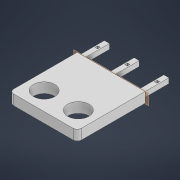
# Autodesk Inventor part: Ultrasonic Mount
Saved by Autodesk Inventor 2022 (Build 260153000, 153)
## iProperties
Created: 2021-06-09
Part Number: Ultrasonic Mount
Material: Generic
Document SubType Name: Modeling
Designer: saatvik123
Density: 1 g/cm^3
Appearance: Default
Author: saatvik123
## iProperties of the stored document Ultrasonic Mount_3DPrint.ipt
Created: 2021-06-09
Part Number: Ultrasonic Mount_3DPrint
Material: Generic
Document SubType Name: Modeling
Designer: saatvik123
Density: 1 g/cm^3
Appearance: Default
Author: saatvik123
Autodesk Inventor part; units mm, degrees
ref_plane "YZ Plane" through (0, 0, 0) normal (1, 0, 0) x (0, 1, 0)
ref_plane "XZ Plane" through (0, 0, 0) normal (0, 1, 0) x (-1, 0, 0)
ref_plane "XY Plane" through (0, 0, 0) normal (0, 0, 1) x (1, 0, 0)
ref_plane "Work Plane1" through (0, 0, 0) normal (0, 0, 1) x (1, 0, 0)
sketch "Sketch1" plane through (0, 0, 0) normal (0, 0, 1) x (1, 0, 0)
  line L0 (24.13, -1.27) -> (20.32, -1.27) projected
  line L1 (20.32, -1.27) -> (20.32, 2.54) projected
  line L2 (20.32, 2.54) -> (24.13, 2.54) projected
  line L3 (24.13, 2.54) -> (24.13, -1.27) projected
  line L4 (-1.905, -1.27) -> (-1.905, 2.54) projected
  line L5 (-1.905, 2.54) -> (1.905, 2.54) projected
  line L6 (1.905, 2.54) -> (1.905, -1.27) projected
  line L7 (1.905, -1.27) -> (-1.905, -1.27) projected
  line L8 (-20.32, 2.54) -> (-20.32, -1.27) projected
  line L9 (-20.32, -1.27) -> (-24.13, -1.27) projected
  line L10 (-24.13, -1.27) -> (-24.13, 2.54) projected
  line L11 (-24.13, 2.54) -> (-20.32, 2.54) projected
  line L12 (-25.4, 3.81) -> (25.4, 3.81) projected
  line L13 (-25.4, -3.81) -> (-25.4, 3.81) projected
  line L14 (25.4, -3.81) -> (-25.4, -3.81) projected
  line L15 (25.4, 3.81) -> (25.4, -3.81) projected
  point P0 (0, 0)
extrude "Extrusion1" add sketch "Sketch1" against normal blind 19.05 contours L0 L1 L2 L3 | L4 L5 L6 L7 | L8 L9 L10 L11
sketch "Sketch2" plane through (-24.13, 2.54, 0) normal (0, 1, 0) x (1, 0, 0)
  line L0 (47.3075, 11.1125) -> (45.4025, 11.1125) projected
  line L1 (45.4025, 11.1125) -> (45.4025, 13.0175) projected
  line L2 (45.4025, 13.0175) -> (47.3075, 13.0175) projected
  line L3 (47.3075, 13.0175) -> (47.3075, 11.1125) projected
  line L4 (23.1775, 13.0175) -> (25.0825, 13.0175) projected
  line L5 (25.0825, 13.0175) -> (25.0825, 11.1125) projected
  line L6 (25.0825, 11.1125) -> (23.1775, 11.1125) projected
  line L7 (23.1775, 11.1125) -> (23.1775, 13.0175) projected
  line L8 (0.9525, 13.0175) -> (2.8575, 13.0175) projected
  line L9 (2.8575, 13.0175) -> (2.8575, 11.1125) projected
  line L10 (2.8575, 11.1125) -> (0.9525, 11.1125) projected
  line L11 (0.9525, 11.1125) -> (0.9525, 13.0175) projected
  point P0 (24.13, 0)
extrude "Extrusion2" cut sketch "Sketch2" against normal blind 3.81
ref_plane "Work Plane2" through (0, 0, 0) normal (0, 0, 1) x (1, 0, 0)
sketch "Sketch3" plane through (0, 0, 0) normal (0, 0, 1) x (1, 0, 0)
  line L0 (24.13, -1.27) -> (20.32, -1.27) projected
  line L1 (20.32, -1.27) -> (20.32, 2.54) projected
  line L2 (20.32, 2.54) -> (24.13, 2.54) projected
  line L3 (24.13, 2.54) -> (24.13, -1.27) projected
  line L4 (-1.905, -1.27) -> (-1.905, 2.54) projected
  line L5 (-1.905, 2.54) -> (1.905, 2.54) projected
  line L6 (1.905, 2.54) -> (1.905, -1.27) projected
  line L7 (1.905, -1.27) -> (-1.905, -1.27) projected
  line L8 (-20.32, 2.54) -> (-20.32, -1.27) projected
  line L9 (-20.32, -1.27) -> (-24.13, -1.27) projected
  line L10 (-24.13, -1.27) -> (-24.13, 2.54) projected
  line L11 (-24.13, 2.54) -> (-20.32, 2.54) projected
  line L12 (-25.4, 3.81) -> (25.4, 3.81) projected
  line L13 (-25.4, -3.81) -> (-25.4, 3.81) projected
  line L14 (25.4, -3.81) -> (-25.4, -3.81) projected
  line L15 (25.4, 3.81) -> (25.4, -3.81) projected
  point P0 (0, 0)
extrude "Extrusion3" add sketch "Sketch3" along normal blind 50.8 contours L0 L1 L2 L3 | L4 L5 L6 L7 | L8 L9 L10 L11 | L12 L15 L14 L13
sketch "Sketch4" plane through (-25.4, 3.81, 0) normal (0, 1, 0) x (1, 0, 0)
  circle A0 centre (12.377, -37.1786) radius 7.95 projected
  circle A1 centre (37.977, -37.1786) radius 7.95 projected
  line L0 (50.8, -50.8) -> (0, -50.8) projected
  point P0 (25.4, 0)
  dimension "d6" = 15.9
  dimension "d7" = 15.9
  dimension "d8" = 13.6214
  measures "d6" diameter of A1
  measures "d7" diameter of A0
  measures "d8" distance from line of L0 A0.centre
extrude "Extrusion4" cut sketch "Sketch4" against normal blind 7.62
fillet "Fillet1" radius 3.175 2 edges at (-25.4, 0, 50.8) (25.4, 0, 50.8)
body "Solid1"
